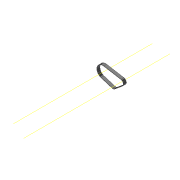
# Autodesk Inventor part: Synchronous Belt
Saved by Autodesk Inventor 2018 (Build 220112000, 112)
## iProperties
Created: 2019-08-30
Part Number: Synchronous Belt
Material: Rubber
Document SubType Name: Modeling
Designer: Clevo
Density: 1 g/cm^3
Appearance: Rubber - Black - Version 1.1
CustomPartVersion: 1
Author: Clevo
Autodesk Inventor part; units mm, degrees
ref_plane "YZ Plane" through (0, 0, 0) normal (1, 0, 0) x (0, 1, 0)
ref_plane "XZ Plane" through (0, 0, 0) normal (0, 1, 0) x (-1, 0, 0)
ref_plane "XY Plane" through (0, 0, 0) normal (0, 0, 1) x (1, 0, 0)
sketch "Sketch Path" plane through (0, 0, 0) normal (0, 0, 1) x (1, 0, 0)
  arc A0 (3.819797, -4.585834) -> (1.021383, 5.880264) centre (0, 0) ccw
  arc A1 (-16.681735, -19.299334) -> (-12.953468, -18.557223) centre (-15.5, -15.5) ccw
  arc A2 (-35.089142, 12.152546) -> (-40.86338, -11.777934) centre (-37.2, 0) ccw
  line L0 (-35.089142, 12.152546) -> (1.021383, 5.880264)
  line L1 (3.819797, -4.585834) -> (-12.953468, -18.557223)
  line L2 (-16.681735, -19.299334) -> (-40.86338, -11.777934)
  constraints: 6 end point, 6 point on circle, 3 centre point
ref_plane "Cross Section Plane" through (1.021383, 5.880264, 0) normal (-0.9852477, 0.1711343, 0) x (0, 0, 1)
ref_plane "Work Plane2" through (0, 0, 0) normal (-1, 0, 0) x (0, 0, 1)
ref_plane "Work Plane3" through (-15.5, -15.5, 0) normal (0.9102985, 0.4139525, 0) x (0, 0, 1)
ref_plane "Work Plane4" through (-37.2, 0, 0) normal (0.9023212, -0.4310643, 0) x (0, 0, 1)
sketch "Cross Section" plane through (1.021383, 5.880264, 0) normal (-0.9852477, 0.1711343, 0) x (0, 0, 1)
  line L0 (-3, 0.3) -> (3, 0.3)
  line L1 (3, 0.3) -> (3, -0.3)
  line L2 (3, -0.3) -> (-3, -0.3)
  line L3 (-3, -0.3) -> (-3, 0.3)
  line L4 (-3, 0) -> (3, 0) construction
  point P0 (0, 0)
  point P1 (0, 0)
  dimension "d0" = 6
  dimension "d4" = 0.3
  dimension "d5" = 0.3
  constraints: 10 end point, 3 midpoint, 2 parallel, 1 coincident, 1 horizontal, 1 perpendicular, 1 other
  measures "d0" distance between parallel lines of L1 L3
  measures "d4" distance between parallel lines of L2 L4
  measures "d5" distance between parallel lines of L4 L0
sweep "Belt" add profiles "Cross Section" path "Sketch Path" path curves L2 A2 L0 A0 L1 A1
equation "\"d0\" = da_B"
equation "\"d4\" = da_a"
equation "\"d5\" = da_a2"
equation "\"da_B\" = 6"
equation "\"da_pb\" = 2.5"
equation "\"da_L\" = 138.49893"
equation "\"da_a\" = 0.3"
equation "\"da_S\" = 1.5"
equation "\"da_Beta\" = 20deg"
equation "\"da_Ht\" = 0.7"
equation "\"da_H\" = 1.3"
equation "\"da_a2\" = 0.3"
body "Solid1"
